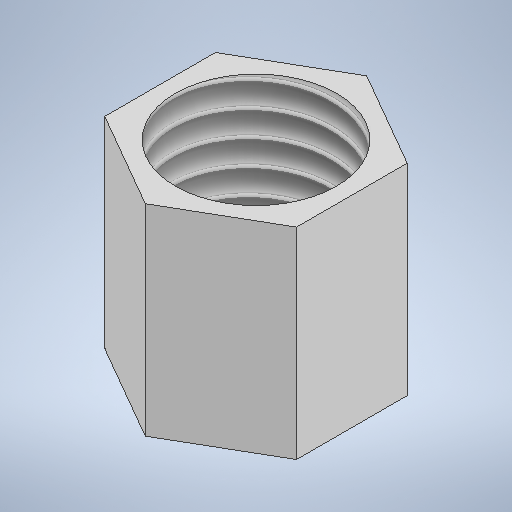
# Autodesk Inventor part: 159
Saved by Autodesk Inventor 2025.1 (Build 291241000, 241)
## iProperties
Created: 2024-08-20
Part Number: 159
Material: Generisch
Document SubType Name: Modeling
Designer: ffogue
Density: 1 g/cm^3
Appearance: Vorgabe
Author: ffogue
Autodesk Inventor part; units mm, degrees
ref_plane "YZ Plane" through (0, 0, 0) normal (1, 0, 0) x (0, 1, 0)
ref_plane "XZ Plane" through (0, 0, 0) normal (0, 1, 0) x (-1, 0, 0)
ref_plane "XY Plane" through (0, 0, 0) normal (0, 0, 1) x (1, 0, 0)
sketch "Sketch1" plane through (0, 0, 0) normal (0, 0, 1) x (1, 0, 0)
  line L0 (0, 5.5) -> (4.7631, 2.75)
  line L1 (4.7631, 2.75) -> (4.7631, -2.75)
  line L2 (4.7631, -2.75) -> (0, -5.5)
  line L3 (0, -5.5) -> (-4.7631, -2.75)
  line L4 (-4.7631, -2.75) -> (-4.7631, 2.75)
  line L5 (-4.7631, 2.75) -> (0, 5.5)
  point P0 (0, 0)
  point P1 (0, 0)
  dimension "d0" = 11
  constraints: 12 end point, 1 coincident, 13 other
  measures "d0" distance of L2.end L0.start
extrude "Extrusion1" add sketch "Sketch1" against normal blind 10
sketch "Sketch3" plane through (0, 0, 0) normal (0, 0, 1) x (1, 0, 0)
  point P0 (0, 0)
  point P1 (0, 0)
  constraints: 1 coincident
hole "Hole1" at (0, 0, 0) direction (0, 0, -1) diameter 8 depth 7
thread "Thread2" size "M8x1.25" class "6H" standard "ISO Metric profile" length 15
sketch "Sketch4" plane through (0, 0, -10) normal (0, 0, -1) x (-1, 0, 0)
  point P0 (0, 0)
  point P1 (0, 0)
  constraints: 1 coincident
hole "Hole2" at (0, 0, -10) direction (0, 0, 1) diameter 5 depth 5
body "Solid1"
